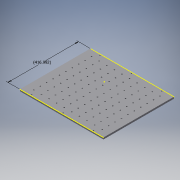
# Autodesk Inventor part: BattleBot-TopPlate-Redesign
Saved by Autodesk Inventor 2017 (Build 210142000, 142)
## iProperties
Created: 2016-09-29
Part Number: BattleBot-TopPlate-Redesign
Material: Generic
Document SubType Name: Modeling
Designer: Adam Popescu
Density: 1 g/cm^3
Appearance: Default
Author: Adam Popescu
Autodesk Inventor part; units mm, degrees
ref_plane "YZ Plane" through (0, 0, 0) normal (1, 0, 0) x (0, 1, 0)
ref_plane "XZ Plane" through (0, 0, 0) normal (0, 1, 0) x (-1, 0, 0)
ref_plane "XY Plane" through (0, 0, 0) normal (0, 0, 1) x (1, 0, 0)
sketch "Sketch1" plane through (0, 0, 0) normal (0, 1, 0) x (-1, 0, 0)
  line L0 (212.1429, -130.4286) -> (-281.8571, -130.4286)
  line L1 (-281.8571, -130.4286) -> (-281.8571, 286.5714)
  line L2 (-281.8571, 286.5714) -> (212.1429, 286.5714)
  line L3 (212.1429, 286.5714) -> (212.1429, -130.4286)
  point P0 (0, 0)
  dimension "d0" = 494
  dimension "d1" = 417
  constraints: 8 end point, 2 parallel, 1 horizontal, 1 perpendicular
  measures "d0" distance of L0.start L0.end
  measures "d1" distance of L2.end L0.start
extrude "Extrusion1" add sketch "Sketch1" along normal blind 10
sketch "Sketch3" plane through (0, 10, 0) normal (0, 1, 0) x (1, 0, 0)
  line L0 (-212.1429, -286.5714) -> (281.8571, -286.5714) projected
  line L1 (281.8571, 130.4286) -> (-212.1429, 130.4286) projected
  point P0 (0, 0)
  dimension "d4" = 416.9918
sketch "Sketch4" plane through (0, 10, 0) normal (0, 1, 0) x (1, 0, 0)
  circle A0 centre (216.8571, -279.5714) radius 3.175
  circle A1 centre (56.7978, -63.9355) radius 3.6308
  circle A2 centre (36.104, -63.9355) radius 3.736
  line L0 (281.8571, 130.4286) -> (-212.1429, 130.4286) projected
  line L1 (281.8571, -286.5714) -> (281.8571, 130.4286) projected
  point P0 (0, 0)
  dimension "d5" = 6.35
  dimension "d6" = 410
  dimension "d7" = 65
  constraints: 3 centre point
  measures "d5" diameter of A0
  measures "d6" distance from line of L0 A0.centre
  measures "d7" distance from line of L1 A0.centre
extrude "Extrusion2" cut sketch "Sketch4" against normal blind 10 contours A0
sketch "Sketch5" plane through (0, 10, 0) normal (0, 1, 0) x (1, 0, 0)
  circle A0 centre (36.8571, -279.5782) radius 3.175
  line L0 (281.8571, 130.4286) -> (-212.1429, 130.4286) projected
  circle A1 centre (216.8571, -279.5714) radius 3.175 projected
  line L1 (281.8571, -286.5714) -> (281.8571, 130.4286) projected
  point P0 (0, 0)
  dimension "d10" = 6.35
  dimension "d11" = 410.0068
  dimension "d12" = 410
  dimension "d13" = 245
  constraints: 1 centre point
  measures "d10" diameter of A0
  measures "d11" distance from line of L0 A0.centre
  measures "d12" distance from line of L0 A1.centre
  measures "d13" distance from line of L1 A0.centre
extrude "Extrusion3" cut sketch "Sketch5" against normal blind 10 contours A0
sketch "Sketch6" plane through (0, 10, 0) normal (0, 1, 0) x (1, 0, 0)
  circle A0 centre (-149.1429, -279.5782) radius 3.175
  line L0 (281.8571, 130.4286) -> (-212.1429, 130.4286) projected
  line L1 (281.8571, -286.5714) -> (281.8571, 130.4286) projected
  point P0 (0, 0)
  dimension "d16" = 6.35
  dimension "d17" = 410.0068
  dimension "d18" = 431
  constraints: 1 centre point
  measures "d16" diameter of A0
  measures "d17" distance from line of L0 A0.centre
  measures "d18" distance from line of L1 A0.centre
extrude "Extrusion4" cut sketch "Sketch6" against normal blind 13.175
sketch "Sketch7" plane through (0, 10, 0) normal (0, 1, 0) x (1, 0, 0)
  circle A0 centre (216.8571, 123.4354) radius 3.175
  line L0 (281.8571, -286.5714) -> (281.8571, 130.4286) projected
  line L1 (-212.1429, -286.5714) -> (281.8571, -286.5714) projected
  point P0 (0, 0)
  dimension "d21" = 6.35
  dimension "d22" = 65
  dimension "d23" = 410.0068
  constraints: 1 centre point
  measures "d21" diameter of A0
  measures "d22" distance from line of L0 A0.centre
  measures "d23" distance from line of L1 A0.centre
extrude "Extrusion5" cut sketch "Sketch7" against normal blind 10
sketch "Sketch8" plane through (0, 10, 0) normal (0, 1, 0) x (1, 0, 0)
  point P0 (0, 0)
sketch "Sketch9" plane through (0, 10, 0) normal (0, 1, 0) x (1, 0, 0)
  circle A0 centre (36.8571, 123.4354) radius 3.175
  line L0 (-212.1429, -286.5714) -> (281.8571, -286.5714) projected
  line L1 (281.8571, -286.5714) -> (281.8571, 130.4286) projected
  point P0 (0, 0)
  dimension "d26" = 6.35
  dimension "d27" = 410.0068
  dimension "d28" = 245
  constraints: 1 centre point
  measures "d26" diameter of A0
  measures "d27" distance from line of L0 A0.centre
  measures "d28" distance from line of L1 A0.centre
extrude "Extrusion6" cut sketch "Sketch9" against normal blind 10
sketch "Sketch10" plane through (0, 10, 0) normal (0, 1, 0) x (1, 0, 0)
  circle A0 centre (-149.1429, 123.4354) radius 3.175
  line L0 (-212.1429, -286.5714) -> (281.8571, -286.5714) projected
  line L1 (281.8571, -286.5714) -> (281.8571, 130.4286) projected
  point P0 (0, 0)
  dimension "d31" = 6.35
  dimension "d32" = 410.0068
  dimension "d33" = 431
  constraints: 1 centre point
  measures "d31" diameter of A0
  measures "d32" distance from line of L0 A0.centre
  measures "d33" distance from line of L1 A0.centre
extrude "Extrusion7" cut sketch "Sketch10" against normal blind 10
sketch "Sketch15" plane through (0, 10, 0) normal (0, 1, 0) x (1, 0, 0)
  line L0 (281.8571, 130.4286) -> (-212.1429, 130.4286) projected
  line L1 (-212.1429, 130.4286) -> (-212.1429, -286.5714) projected
  circle A0 centre (-167.2339, 92.5206) radius 3.5
  circle A1 centre (-122.3249, 92.5206) radius 3.5
  circle A2 centre (-77.4159, 92.5206) radius 3.5
  circle A3 centre (-32.5069, 92.5206) radius 3.5
  circle A4 centre (12.4021, 92.5206) radius 3.5
  circle A5 centre (57.3111, 92.5206) radius 3.5
  circle A6 centre (102.2201, 92.5206) radius 3.5
  circle A7 centre (147.1291, 92.5206) radius 3.5
  circle A8 centre (192.0381, 92.5206) radius 3.5
  circle A9 centre (236.9471, 92.5206) radius 3.5
  circle A10 centre (-167.2339, 54.6126) radius 3.5
  circle A11 centre (-122.3249, 54.6126) radius 3.5
  circle A12 centre (-77.4159, 54.6126) radius 3.5
  circle A13 centre (-32.5069, 54.6126) radius 3.5
  circle A14 centre (12.4021, 54.6126) radius 3.5
  circle A15 centre (57.3111, 54.6126) radius 3.5
  circle A16 centre (102.2201, 54.6126) radius 3.5
  circle A17 centre (147.1291, 54.6126) radius 3.5
  circle A18 centre (192.0381, 54.6126) radius 3.5
  circle A19 centre (236.9471, 54.6126) radius 3.5
  circle A20 centre (-167.2339, 16.7046) radius 3.5
  circle A21 centre (-122.3249, 16.7046) radius 3.5
  circle A22 centre (-77.4159, 16.7046) radius 3.5
  circle A23 centre (-32.5069, 16.7046) radius 3.5
  circle A24 centre (12.4021, 16.7046) radius 3.5
  circle A25 centre (57.3111, 16.7046) radius 3.5
  circle A26 centre (102.2201, 16.7046) radius 3.5
  circle A27 centre (147.1291, 16.7046) radius 3.5
  circle A28 centre (192.0381, 16.7046) radius 3.5
  circle A29 centre (236.9471, 16.7046) radius 3.5
  circle A30 centre (-167.2339, -21.2034) radius 3.5
  circle A31 centre (-122.3249, -21.2034) radius 3.5
  circle A32 centre (-77.4159, -21.2034) radius 3.5
  circle A33 centre (-32.5069, -21.2034) radius 3.5
  circle A34 centre (12.4021, -21.2034) radius 3.5
  circle A35 centre (57.3111, -21.2034) radius 3.5
  circle A36 centre (102.2201, -21.2034) radius 3.5
  circle A37 centre (147.1291, -21.2034) radius 3.5
  circle A38 centre (192.0381, -21.2034) radius 3.5
  circle A39 centre (236.9471, -21.2034) radius 3.5
  circle A40 centre (-167.2339, -59.1114) radius 3.5
  circle A41 centre (-122.3249, -59.1114) radius 3.5
  circle A42 centre (-77.4159, -59.1114) radius 3.5
  circle A43 centre (-32.5069, -59.1114) radius 3.5
  circle A44 centre (12.4021, -59.1114) radius 3.5
  circle A45 centre (57.3111, -59.1114) radius 3.5
  circle A46 centre (102.2201, -59.1114) radius 3.5
  circle A47 centre (147.1291, -59.1114) radius 3.5
  circle A48 centre (192.0381, -59.1114) radius 3.5
  circle A49 centre (236.9471, -59.1114) radius 3.5
  circle A50 centre (-167.2339, -97.0194) radius 3.5
  circle A51 centre (-122.3249, -97.0194) radius 3.5
  circle A52 centre (-77.4159, -97.0194) radius 3.5
  circle A53 centre (-32.5069, -97.0194) radius 3.5
  circle A54 centre (12.4021, -97.0194) radius 3.5
  circle A55 centre (57.3111, -97.0194) radius 3.5
  circle A56 centre (102.2201, -97.0194) radius 3.5
  circle A57 centre (147.1291, -97.0194) radius 3.5
  circle A58 centre (192.0381, -97.0194) radius 3.5
  circle A59 centre (236.9471, -97.0194) radius 3.5
  circle A60 centre (-167.2339, -134.9274) radius 3.5
  circle A61 centre (-122.3249, -134.9274) radius 3.5
  circle A62 centre (-77.4159, -134.9274) radius 3.5
  circle A63 centre (-32.5069, -134.9274) radius 3.5
  circle A64 centre (12.4021, -134.9274) radius 3.5
  circle A65 centre (57.3111, -134.9274) radius 3.5
  circle A66 centre (102.2201, -134.9274) radius 3.5
  circle A67 centre (147.1291, -134.9274) radius 3.5
  circle A68 centre (192.0381, -134.9274) radius 3.5
  circle A69 centre (236.9471, -134.9274) radius 3.5
  circle A70 centre (-167.2339, -172.8354) radius 3.5
  circle A71 centre (-122.3249, -172.8354) radius 3.5
  circle A72 centre (-77.4159, -172.8354) radius 3.5
  circle A73 centre (-32.5069, -172.8354) radius 3.5
  circle A74 centre (12.4021, -172.8354) radius 3.5
  circle A75 centre (57.3111, -172.8354) radius 3.5
  circle A76 centre (102.2201, -172.8354) radius 3.5
  circle A77 centre (147.1291, -172.8354) radius 3.5
  circle A78 centre (192.0381, -172.8354) radius 3.5
  circle A79 centre (236.9471, -172.8354) radius 3.5
  circle A80 centre (-167.2339, -210.7434) radius 3.5
  circle A81 centre (-122.3249, -210.7434) radius 3.5
  circle A82 centre (-77.4159, -210.7434) radius 3.5
  circle A83 centre (-32.5069, -210.7434) radius 3.5
  circle A84 centre (12.4021, -210.7434) radius 3.5
  circle A85 centre (57.3111, -210.7434) radius 3.5
  circle A86 centre (102.2201, -210.7434) radius 3.5
  circle A87 centre (147.1291, -210.7434) radius 3.5
  circle A88 centre (192.0381, -210.7434) radius 3.5
  circle A89 centre (236.9471, -210.7434) radius 3.5
  circle A90 centre (-167.2339, -248.6514) radius 3.5
  circle A91 centre (-122.3249, -248.6514) radius 3.5
  circle A92 centre (-77.4159, -248.6514) radius 3.5
  circle A93 centre (-32.5069, -248.6514) radius 3.5
  circle A94 centre (12.4021, -248.6514) radius 3.5
  circle A95 centre (57.3111, -248.6514) radius 3.5
  circle A96 centre (102.2201, -248.6514) radius 3.5
  circle A97 centre (147.1291, -248.6514) radius 3.5
  circle A98 centre (192.0381, -248.6514) radius 3.5
  circle A99 centre (236.9471, -248.6514) radius 3.5
  point P0 (0, 0)
  dimension "d130" = 7
  dimension "d131" = 37.908
  dimension "d132" = 44.909
  dimension "d135" = 44.909
  dimension "d138" = 37.908
  constraints: 100 centre point, 1 horizontal, 1 vertical, 198 other
  measures "d130" diameter of A0
  measures "d131" distance from line of L0 A0.centre
  measures "d132" distance from line of L1 A0.centre
  measures "d135" distance of A0.centre A1.centre
  measures "d138" distance of A0.centre A10.centre
extrude "Extrusion10" cut sketch "Sketch15" against normal through all
body "Solid1"
